Autodesk Fusion 360 part; units mm, degrees
(part 3 of 3)
combine "Combine2'" operation add target body 92 tool bodies 94 in component "Chute B left"
sketch "Dropper floor clearance cut sketch" plane through (0, 0, 0) normal (0, 0, 1) x (1, 0, 0) in component "Chute B left"
  circle A0 centre (0, 0) radius 140
extrude "Dropper floor clearance cut" cut sketch "Dropper floor clearance cut sketch" along normal blind 10 from surface at 87 bodies 92 in component "Chute B left"
sketch "Trim sketch" plane through (0, 0, 0) normal (0, 0, 1) x (1, 0, 0) in component "Chute B left"
  circle A0 centre (0, 0) radius 140
  circle A1 centre (0, 0) radius 105
extrude "Trim" add sketch "Trim sketch" along normal blind 70 from surface at 20 separate body makes body 95 in component "Chute B left"
combine "Combine3" operation cut target body 92 tool bodies 95 in component "Chute B left"
sketch "Hopper sketch (2)" plane through (0, 0, 0) normal (0, 0, 1) x (1, 0, 0) in component "Hopper A right"
  line L0 (-47.2943, -42.8507) -> (-31.738, -27.2943)
  line L1 (-31.738, -27.2943) -> (-47.2943, -11.738)
  line L2 (-47.2943, -11.738) -> (-62.8507, -27.2943)
  line L3 (-62.8507, -27.2943) -> (-47.2943, -42.8507)
extrude "Hopper'" add sketch "Hopper sketch (2)" along normal blind 15 from surface at 72 separate body makes body 96 in component "Hopper A right"
sketch "Hopper flange sketch (2)" plane through (0, 0, 0) normal (0, 0, 1) x (1, 0, 0) in component "Hopper A right"
  line L0 (-47.2943, -45.6791) -> (-28.9095, -27.2943)
  line L1 (-28.9095, -27.2943) -> (-47.2943, -8.9095)
  line L2 (-47.2943, -8.9095) -> (-65.6791, -27.2943)
  line L3 (-65.6791, -27.2943) -> (-47.2943, -45.6791)
extrude "Hopper flange'" add sketch "Hopper flange sketch (2)" along normal blind 1.5 from surface at 85.5 bodies 96 in component "Hopper A right"
sketch "Hopper void sketch (2)" plane through (0, 0, 0) normal (0, 0, 1) x (1, 0, 0) in component "Hopper A right"
  line L0 (-47.2943, -38.608) -> (-35.9806, -27.2943)
  line L1 (-35.9806, -27.2943) -> (-47.2943, -15.9806)
  line L2 (-47.2943, -15.9806) -> (-58.608, -27.2943)
  line L3 (-58.608, -27.2943) -> (-47.2943, -38.608)
extrude "Hopper void'" cut sketch "Hopper void sketch (2)" along normal blind 14.4 from surface at 73.6 bodies 96 in component "Hopper A right"
sketch "Socket tool sketch (2)" plane through (0, 0, 0) normal (0, 0, 1) x (1, 0, 0) in component "Hopper A right"
  line L0 (-10.6, -9.6) -> (10.6, -9.6)
  line L1 (10.6, -9.6) -> (10.6, 19.6)
  line L2 (10.6, 19.6) -> (-10.6, 19.6)
  line L3 (-10.6, 19.6) -> (-10.6, -9.6)
extrude "Socket tool'" add sketch "Socket tool sketch (2)" along normal blind 35 separate body makes body 97 in component "Hopper A right"
move_body "Move1'''" bodies 97 to x (0.977496, -0.210954, 0) y (-0.112564, -0.521586, 0.845741) z (-0.178413, -0.826708, -0.533594) at (-46.4023, -23.1608, 82.168) in component "Hopper A right"
combine "Combine1'''" operation cut target body 96 tool bodies 97 in component "Hopper A right"
sketch "Channel sketch (2)" plane through (0, 0, 0) normal (0, 0, 1) x (1, 0, 0) in component "Chute A right"
  line L0 (-10.6, -9.6) -> (10.6, -9.6)
  line L1 (10.6, -9.6) -> (10.6, 11.6)
  line L2 (10.6, 11.6) -> (-10.6, 11.6)
  line L3 (-10.6, 11.6) -> (-10.6, -9.6)
extrude "Channel'" add sketch "Channel sketch (2)" along normal blind 79.2151 separate body makes body 98 in component "Chute A right"
move_body "Move1''''" bodies 98 to x (0.977496, -0.210954, 0) y (-0.112564, -0.521586, 0.845741) z (-0.178413, -0.826708, -0.533594) at (-47.2943, -27.2943, 79.5) in component "Chute A right"
sketch "Channel void sketch (2)" plane through (0, 0, 0) normal (0, 0, 1) x (1, 0, 0) in component "Chute A right"
  line L0 (-9, -8) -> (9, -8)
  line L1 (9, -8) -> (9, 10)
  line L2 (9, 10) -> (-9, 10)
  line L3 (-9, 10) -> (-9, -8)
extrude "Channel void'" add sketch "Channel void sketch (2)" along normal blind 83.2151 separate body makes body 99 in component "Chute A right"
move_body "Move2''" bodies 99 to x (0.977496, -0.210954, 0) y (-0.112564, -0.521586, 0.845741) z (-0.178413, -0.826708, -0.533594) at (-46.9375, -25.6409, 80.5672) in component "Chute A right"
combine "Combine1''''" operation cut target body 98 tool bodies 99 in component "Chute A right"
sketch "Trough cut sketch (2)" plane through (0, 0, 0) normal (0, 0, 1) x (1, 0, 0) in component "Chute A right"
  line L0 (-47.2943, -44.972) -> (-29.6167, -27.2943)
  line L1 (-29.6167, -27.2943) -> (-47.2943, -9.6167)
  line L2 (-47.2943, -9.6167) -> (-64.972, -27.2943)
  line L3 (-64.972, -27.2943) -> (-47.2943, -44.972)
extrude "Trough cut'" cut sketch "Trough cut sketch (2)" along normal blind 40 from surface at 50 bodies 98 in component "Chute A right"
sketch "Floor slab sketch (2)" plane through (0, 0, 0) normal (0, 0, 1) x (1, 0, 0) in component "Chute A right"
  line L0 (-10.6, -9.6) -> (10.6, -9.6)
  line L1 (10.6, -9.6) -> (10.6, -8)
  line L2 (10.6, -8) -> (-10.6, -8)
  line L3 (-10.6, -8) -> (-10.6, -9.6)
extrude "Floor slab'" add sketch "Floor slab sketch (2)" along normal blind 28 separate body makes body 100 in component "Chute A right"
move_body "Move3'" bodies 100 to x (0.977496, -0.210954, 0) y (-0.112564, -0.521586, 0.845741) z (-0.178413, -0.826708, -0.533594) at (-47.2943, -27.2943, 79.5) in component "Chute A right"
combine "Combine2''" operation add target body 98 tool bodies 100 in component "Chute A right"
sketch "Dropper floor clearance cut sketch (2)" plane through (0, 0, 0) normal (0, 0, 1) x (1, 0, 0) in component "Chute A right"
  circle A0 centre (0, 0) radius 140
extrude "Dropper floor clearance cut'" cut sketch "Dropper floor clearance cut sketch (2)" along normal blind 10 from surface at 87 bodies 98 in component "Chute A right"
sketch "Trim sketch (2)" plane through (0, 0, 0) normal (0, 0, 1) x (1, 0, 0) in component "Chute A right"
  circle A0 centre (0, 0) radius 140
  circle A1 centre (0, 0) radius 105
extrude "Trim'" add sketch "Trim sketch (2)" along normal blind 70 from surface at 20 separate body makes body 101 in component "Chute A right"
combine "Combine3'" operation cut target body 98 tool bodies 101 in component "Chute A right"
component "Tub" placed x (1, 0, 0) y (0, 1, 0) z (0, 0, 1) at (0, 0, 0)
component "Wheel L" placed x (1, 0, 0) y (0, 1, 0) z (0, 0, 1) at (0, 0, 0)
component "Motor L" placed x (1, 0, 0) y (0, 1, 0) z (0, 0, 1) at (0, 0, 0)
component "Wheel R" placed x (1, 0, 0) y (0, 1, 0) z (0, 0, 1) at (0, 0, 0)
component "Motor R" placed x (1, 0, 0) y (0, 1, 0) z (0, 0, 1) at (0, 0, 0)
component "Face plate L" placed x (1, 0, 0) y (0, 1, 0) z (0, 0, 1) at (0, 0, 0)
component "Face plate R" placed x (1, 0, 0) y (0, 1, 0) z (0, 0, 1) at (0, 0, 0)
component "Omni wheel" placed x (1, 0, 0) y (0, 1, 0) z (0, 0, 1) at (0, 0, 0)
component "Omni arm" placed x (1, 0, 0) y (0, 1, 0) z (0, 0, 1) at (0, 0, 0)
component "Omni pins" placed x (1, 0, 0) y (0, 1, 0) z (0, 0, 1) at (0, 0, 0)
component "Rear nub" placed x (1, 0, 0) y (0, 1, 0) z (0, 0, 1) at (0, 0, 0)
component "Bumper L" placed x (1, 0, 0) y (0, 1, 0) z (0, 0, 1) at (0, 0, 0)
component "Bumper switch L" placed x (1, 0, 0) y (0, 1, 0) z (0, 0, 1) at (0, 0, 0)
component "Bumper R" placed x (1, 0, 0) y (0, 1, 0) z (0, 0, 1) at (0, 0, 0)
component "Bumper switch R" placed x (1, 0, 0) y (0, 1, 0) z (0, 0, 1) at (0, 0, 0)
component "Upper frame" placed x (1, 0, 0) y (0, 1, 0) z (0, 0, 1) at (0, 0, 0)
component "ToF F" placed x (1, 0, 0) y (0, 1, 0) z (0, 0, 1) at (0, 0, 0)
component "ToF FL" placed x (1, 0, 0) y (0, 1, 0) z (0, 0, 1) at (0, 0, 0)
component "ToF FR" placed x (1, 0, 0) y (0, 1, 0) z (0, 0, 1) at (0, 0, 0)
component "ToF SFL" placed x (1, 0, 0) y (0, 1, 0) z (0, 0, 1) at (0, 0, 0)
component "ToF SFR" placed x (1, 0, 0) y (0, 1, 0) z (0, 0, 1) at (0, 0, 0)
component "ToF SRL" placed x (1, 0, 0) y (0, 1, 0) z (0, 0, 1) at (0, 0, 0)
component "ToF SRR" placed x (1, 0, 0) y (0, 1, 0) z (0, 0, 1) at (0, 0, 0)
component "ToF RL" placed x (1, 0, 0) y (0, 1, 0) z (0, 0, 1) at (0, 0, 0)
component "ToF RR" placed x (1, 0, 0) y (0, 1, 0) z (0, 0, 1) at (0, 0, 0)
component "Camera L" placed x (1, 0, 0) y (0, 0.34202, 0.939693) z (0, -0.939693, 0.34202) at (3.0712, 87.9464, 93)
component "Camera R" placed x (-1, 0, 0) y (0, -0.34202, 0.939693) z (0, 0.939693, 0.34202) at (3.0712, -87.9464, 93)
component "Lid" placed x (1, 0, 0) y (0, 1, 0) z (0, 0, 1) at (0, 0, 0)
component "Handle bar" placed x (1, 0, 0) y (0, 1, 0) z (0, 0, 1) at (0, 0, 0)
component "Victim LED" placed x (1, 0, 0) y (0, 1, 0) z (0, 0, 1) at (0, 0, 0)
component "Start button" placed x (1, 0, 0) y (0, 1, 0) z (0, 0, 1) at (0, 0, 0)
component "Power switch" placed x (1, 0, 0) y (0, 1, 0) z (0, 0, 1) at (0, 0, 0)
component "Status LED 1" placed x (1, 0, 0) y (0, 1, 0) z (0, 0, 1) at (0, 0, 0)
component "Status LED 2" placed x (1, 0, 0) y (0, 1, 0) z (0, 0, 1) at (0, 0, 0)
component "USB-C service socket" placed x (1, 0, 0) y (0, 1, 0) z (0, 0, 1) at (0, 0, 0)
component "Dropper floor" placed x (1, 0, 0) y (0, 1, 0) z (0, 0, 1) at (0, 0, 0)
component "Dropper plate" placed x (1, 0, 0) y (0, 1, 0) z (0, 0, 1) at (0, 0, 0)
component "N20 motor" placed x (1, 0, 0) y (0, 1, 0) z (0, 0, 1) at (0, 0, 0)
component "N20 face plate" placed x (1, 0, 0) y (0, 1, 0) z (0, 0, 1) at (0, 0, 0)
component "Kits" placed x (1, 0, 0) y (0, 1, 0) z (0, 0, 1) at (0, 0, 0)
component "GIGA posts" placed x (1, 0, 0) y (0, 1, 0) z (0, 0, 1) at (0, 0, 0)
component "Arduino GIGA R1" placed x (1, 0, 0) y (0, 1, 0) z (0, 0, 1) at (0, 0, 0)
component "Main PCB" placed x (1, 0, 0) y (0, 1, 0) z (0, 0, 1) at (0, 0, 0)
component "Battery" placed x (1, 0, 0) y (0, 1, 0) z (0, 0, 1) at (0, 0, 0)
component "Floor port FP" placed x (1, 0, 0) y (0, 1, 0) z (0, 0, 1) at (0, 0, 0)
component "Silver module SM" placed x (1, 0, 0) y (0, 1, 0) z (0, 0, 1) at (0, 0, 0)
component "Wi-Fi antenna" placed x (1, 0, 0) y (0, 1, 0) z (0, 0, 1) at (0, 0, 0)
component "Stepper bay 28BYJ-48" placed x (1, 0, 0) y (0, 1, 0) z (0, 0, 1) at (0, 0, 0)
component "Hopper B left" placed x (1, 0, 0) y (0, 1, 0) z (0, 0, 1) at (0, 0, 0)
component "Chute B left" placed x (1, 0, 0) y (0, 1, 0) z (0, 0, 1) at (0, 0, 0)
component "Hopper A right" placed x (1, 0, 0) y (0, 1, 0) z (0, 0, 1) at (0, 0, 0)
component "Chute A right" placed x (1, 0, 0) y (0, 1, 0) z (0, 0, 1) at (0, 0, 0)
named bodies: "Tub shell", "Chute hole tool B left", "Chute hole tool A right", "Cradle prong front L", "Cradle prong rear L", "Cradle prong front R", "Cradle prong rear R", "Wheel L", "Encoder L", "Gearmotor L", "Motor shaft L", "Wheel R", "Encoder R", "Gearmotor R", "Motor shaft R", "Face plate L", "Face plate R", "Omni wheel", "Arm plate", "Pivot pin", "Axle pin", "Rear nub", "Bumper plate L", "Microswitch L", "Bumper plate R", "Microswitch R", "Frame ring", "VL53L0X module F", "VL53L0X chip F", "VL53L0X module FL", "VL53L0X chip FL", "VL53L0X module FR", "VL53L0X chip FR", "VL53L0X module SFL", "VL53L0X chip SFL", "VL53L0X module SFR", "VL53L0X chip SFR", "VL53L0X module SRL", "VL53L0X chip SRL", "VL53L0X module SRR", "VL53L0X chip SRR", "VL53L0X module RL", "VL53L0X chip RL", "VL53L0X module RR", "VL53L0X chip RR", "Lens block L", "OpenMV H7 Plus board L", "Lens block R", "OpenMV H7 Plus board R", "Lid plate", "Hook bump +71", "Hook bump +114", "Hook bump -71", "Hook bump -114", "Handle bar", "Victim LED", "Start button", "Power switch", "Status LED 1", "Status LED 2", "USB-C service socket", "Dropper floor", "Dropper plate", "N20 gearmotor with encoder", "N20 shaft", "N20 face plate", "Kit 1", "Kit 2", "Kit 3", "Kit 4", "Kit 5", "Kit 6", "Kit 7", "Kit 8", "GIGA post H1", "GIGA post H2", "GIGA post H3", "GIGA post H4", "GIGA board", "Header strip +y", "Header strip -y", "Main PCB shield (placeholder)", "PCB component envelope (placeholder)", "Battery (placeholder 7.0 x 3.5 x 2.5)", "Floor sensor FP (black, blue, red)", "Silver module SM (straight + 20 deg tilted pair)", "USB-C J12", "Wi-Fi antenna", "Body", "Hopper", "Socket tool", "Channel", "Channel void", "Floor slab", "Trim"
